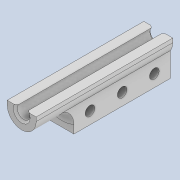
# Autodesk Inventor part: bw_hl_1
Saved by Autodesk Inventor 2020 (Build 240168000, 168)
## iProperties
Created: 2021-09-10
Part Number: bw_hl_1
Material: Generic
Document SubType Name: Modeling
Designer: Shuang Peng
Density: 1 g/cm^3
Appearance: Default
Author: Shuang Peng
Autodesk Inventor part; units mm, degrees
ref_plane "YZ Plane" through (0, 0, 0) normal (1, 0, 0) x (0, 1, 0)
ref_plane "XZ Plane" through (0, 0, 0) normal (0, 1, 0) x (-1, 0, 0)
ref_plane "XY Plane" through (0, 0, 0) normal (0, 0, 1) x (1, 0, 0)
sketch "Sketch1" plane through (0, 0, 0) normal (0, 0, 1) x (1, 0, 0)
  circle A0 centre (0, 0) radius 0.8 projected
  circle A1 centre (0, 0) radius 0.8
  circle A2 centre (0, 0) radius 1.8
  line L0 (0, 0) -> (0, 0.5)
  line L1 (0, 0) -> (-1.8, 0)
  line L2 (0, 0) -> (-1.8, 0)
  line L3 (-1.8, 0) -> (-1.8, 0.5)
  line L4 (-1.8, 0.5) -> (0, 0.5)
  line L5 (0, 0.5) -> (0, 0)
  line L6 (0, 0) -> (1.8, 0)
  line L7 (1.8, 0) -> (1.8, 0.5)
  line L8 (1.8, 0.5) -> (0, 0.5)
  line L9 (0, 0.5) -> (0, 0)
  point P0 (1.8, 0)
  point P1 (0.6245, 0.5)
  point P2 (-0.6245, 0.5)
  dimension "d0" = 1.6
  dimension "d1" = 1
  dimension "d2" = 0.5
  dimension "d3" = 1.8
  dimension "d4" = 0.5
  dimension "d5" = 1.8
  dimension "d6" = 0.5
  constraints: 20 end point, 4 parallel, 3 horizontal, 2 coincident, 2 perpendicular, 1 centre point, 1 vertical, 3 other
  measures "d0" diameter of A1
  measures "d2" distance of L0.start L0.end
  measures "d3" distance of L3.end L4.end
  measures "d4" distance of L2.end L3.end
  measures "d5" distance of L8.end L7.end
  measures "d6" distance of L7.end L6.end
extrude "Extrusion1" add sketch "Sketch1" against normal blind 12 contours L6 A2 L1 A0 | A0 L8 A2 L6 | L1 A2 L4 A0 | A2 L8 L7 | L3 L4 A2
sketch "Sketch2" plane through (0, 0, -12) normal (0, 0, -1) x (-1, 0, 0)
  line L0 (1.8, 0.5) -> (0.6245, 0.5) projected
  arc A0 (-0.6245, 0.5) -> (0.6245, 0.5) centre (0, 0) ccw projected
  line L1 (-0.6245, 0.5) -> (-1.8, 0.5) projected
  line L2 (-1.8, 0.5) -> (-1.8, 0) projected
  arc A1 (-1.8, 0) -> (1.8, 0) centre (0, 0) ccw projected
  line L3 (1.8, 0) -> (1.8, 0.5) projected
  line L4 (0, 0) -> (0, -7)
  line L5 (1.5, 0) -> (-1.5, 0)
  line L6 (-1.5, 0) -> (-1.5, -7)
  line L7 (-1.5, -7) -> (1.5, -7)
  line L8 (1.5, -7) -> (1.5, 0)
  line L9 (1.5, 0) -> (-1.5, -7) construction
  line L10 (-1.5, 0) -> (1.5, -7) construction
  point P0 (0, -3.5)
  point P1 (1.5, -0.995)
  point P2 (-1.5, -0.995)
  dimension "d9" = 7
  dimension "d10" = 3
  dimension "d11" = 7
  constraints: 14 end point, 3 midpoint, 2 parallel, 2 perpendicular, 1 vertical
  measures "d9" distance of L4.start L4.end
  measures "d10" distance of L5.start L5.end
  measures "d11" distance of L6.end L5.end
extrude "Extrusion2" add sketch "Sketch2" against normal blind 12 contours L8 L7 L4 A1 | L4 L7 L6 A1
sketch "Sketch3" plane through (1.5, -7, -12) normal (1, 0, 0) x (0, 0, -1)
  line L0 (0, 3) -> (-13.2788, 3) projected
  line L1 (0, 6.005) -> (0, 0) projected
  line L2 (-12, 6.005) -> (0, 6.005) projected
  line L3 (-12, 0) -> (-12, 6.005) projected
  line L4 (0, 0) -> (-12, 0) projected
  line L5 (-12, 6.005) -> (-12, 3.005)
  line L6 (-12, 6.005) -> (-12, 0) projected
  line L7 (-12, 6.005) -> (-12, 4.505)
  line L8 (-12, 0) -> (-12, 6.005) projected
  line L9 (-12, 4.505) -> (0, 4.505)
  circle A0 centre (-6, 4.505) radius 0.6
  line L10 (-6, 4.505) -> (-10, 4.505)
  circle A1 centre (-10, 4.505) radius 0.6
  line L11 (-6, 4.505) -> (-2, 4.505)
  circle A2 centre (-2, 4.505) radius 0.6
  point P0 (-12, 7)
  dimension "d14" = 3
  dimension "d15" = 1.5
  dimension "d16" = 1.2
  dimension "d17" = 4
  dimension "d18" = 1.2
  dimension "d19" = 4
  dimension "d20" = 1.2
  constraints: 10 end point, 4 point on line, 3 centre point, 2 coincident, 1 collinear, 1 midpoint, 1 perpendicular
  measures "d14" distance of L2.start L5.end
  measures "d15" distance of L2.start L7.end
  measures "d16" diameter of A0
  measures "d17" distance of L10.start L10.end
  measures "d18" diameter of A1
  measures "d19" distance of L10.start L11.end
  measures "d20" diameter of A2
extrude "Extrusion3" cut sketch "Sketch3" against normal blind 12 contours A2 L9 | L9 A2 | A1 L9 | L9 A1 | A0 L9 | L9 A0
sketch "Sketch4" plane through (1.5, -7, -12) normal (1, 0, 0) x (0, 0, -1)
  circle A0 centre (-2, 4.505) radius 0.6 projected
  circle A1 centre (-6, 4.505) radius 0.6 projected
  circle A2 centre (-10, 4.505) radius 0.6 projected
  line L0 (0, 6.005) -> (0, 0) projected
  line L1 (-12, 6.005) -> (0, 6.005) projected
  line L2 (-12, 0) -> (-12, 6.005) projected
  line L3 (0, 0) -> (-12, 0) projected
  line L4 (0, 6.005) -> (-12, 6.005) projected
  line L5 (-12, 6.005) -> (-12, 3.005)
  line L6 (-12, 0) -> (-12, 6.005) projected
  line L7 (-12, 3.005) -> (0, 3.005)
  line L8 (0, 6.005) -> (0, 0) projected
  point P0 (-12, 7)
  dimension "d23" = 3
  constraints: 4 end point, 2 point on line, 1 perpendicular
  measures "d23" distance of L1.start L5.end
extrude "Extrusion4" cut sketch "Sketch4" against normal blind 12 contours L0 L3 L2 L7
sketch "Sketch5" plane through (0, 0, 0) normal (0, 0, 1) x (1, 0, 0)
  line L0 (-1.5, -3.995) -> (1.5, -3.995) projected
  line L1 (1.5, -3.995) -> (1.5, -0.995) projected
  arc A0 (1.5, -0.995) -> (1.8, 0) centre (0, 0) ccw projected
  line L2 (1.8, 0) -> (1.8, 0.5) projected
  line L3 (1.8, 0.5) -> (0.6245, 0.5) projected
  arc A1 (-0.6245, 0.5) -> (0.6245, 0.5) centre (0, 0) ccw projected
  line L4 (-0.6245, 0.5) -> (-1.8, 0.5) projected
  line L5 (-1.8, 0.5) -> (-1.8, 0) projected
  arc A2 (-1.8, 0) -> (-1.5, -0.995) centre (0, 0) ccw projected
  line L6 (-1.5, -0.995) -> (-1.5, -3.995) projected
  circle A3 centre (0, 0) radius 1.8
  point P0 (-1.5, -0.995)
  point P1 (1.5, -0.995)
  dimension "d26" = 3.6
  constraints: 1 centre point, 1 coincident
  measures "d26" diameter of A3
extrude "Extrusion5" add sketch "Sketch5" along normal blind 5 contours A2 A3 L4 A1 L3 A0 | L5 L4 A3 | A3 L3 L2
fillet "Fillet1" radius 1.5 1 edges at (0, -1.8, 0)
chamfer "Chamfer1" distance 0.25 angle 45 2 edges at (0, -0.8, 5) (0, -0.8, -12)
body "Solid1"
